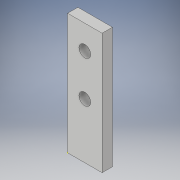
# Autodesk Inventor part: servoPipeConnection
Saved by Autodesk Inventor 2017 (Build 210142000, 142)
## iProperties
Created: 2017-04-06
Part Number: servoPipeConnection
Material: Generic
Document SubType Name: Modeling
Designer: s4461999
Density: 1 g/cm^3
Appearance: Default
Author: s4461999
Autodesk Inventor part; units mm, degrees
ref_plane "YZ Plane" through (0, 0, 0) normal (1, 0, 0) x (0, 1, 0)
ref_plane "XZ Plane" through (0, 0, 0) normal (0, 1, 0) x (-1, 0, 0)
ref_plane "XY Plane" through (0, 0, 0) normal (0, 0, 1) x (1, 0, 0)
sketch "Sketch1" plane through (0, 0, 0) normal (0, 0, 1) x (1, 0, 0)
  line L0 (0, 0) -> (10, 0)
  line L1 (10, 0) -> (10, 35)
  line L2 (10, 35) -> (0, 35)
  line L3 (0, 35) -> (0, 0)
  dimension "d0" = 10
  dimension "d1" = 35
  constraints: 8 end point, 2 parallel, 1 horizontal, 1 perpendicular
  measures "d0" distance of L1.end L2.end
  measures "d1" distance of L2.end L0.start
extrude "Extrusion1" add sketch "Sketch1" along normal blind 3
sketch "Sketch2" plane through (0, 0, 3) normal (0, 0, 1) x (1, 0, 0)
  line L0 (10, 35) -> (0, 35) projected
  line L1 (0, 35) -> (0, 0) projected
  point P0 (5, 28)
  point P1 (5, 16)
  dimension "d4" = 7
  dimension "d5" = 5
  dimension "d6" = 12
  dimension "d7" = 5
  measures "d4" distance from line of L0 point (5, 28)
  measures "d5" distance from line of point (5, 28) L1
  measures "d6" distance of point (5, 28) point (5, 16)
  measures "d7" distance from line of L1 point (5, 16)
hole "Hole1" at (5, 28, 3) at (5, 16, 3) direction (0, 0, -1) diameter 3.4 end through all
sketch "Sketch3" plane through (0, 0, 3) normal (0, 0, 1) x (1, 0, 0)
  point P0 (0, 0)
sketch "Sketch4" plane through (0, 0, 3) normal (0, 0, 1) x (1, 0, 0)
  point P0 (0, 0)
body "Solid1"
